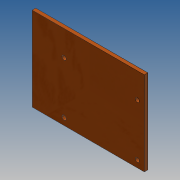
# Autodesk Inventor part: placa circuito
Saved by Autodesk Inventor 2017 (Build 210142000, 142)
## iProperties
Part Number: placa circuito
Material: Genérico
Document SubType Name: Modeling
Designer: Leo
Density: 1 g/cm^3
Appearance: Suave - Naranja claro
Author: Leo
Autodesk Inventor part; units mm, degrees
ref_plane "YZ Plane" through (0, 0, 0) normal (1, 0, 0) x (0, 1, 0)
ref_plane "XZ Plane" through (0, 0, 0) normal (0, 1, 0) x (-1, 0, 0)
ref_plane "XY Plane" through (0, 0, 0) normal (0, 0, 1) x (1, 0, 0)
sketch "Boceto1" plane through (0, 0, 0) normal (0, 1, 0) x (-1, 0, 0)
  line L0 (20, 30) -> (-76, 30)
  line L1 (-76, 30) -> (-76, -30)
  line L2 (-76, -30) -> (20, -30)
  line L3 (20, -30) -> (20, 30)
  line L4 (-3, -25) -> (-58, -25) construction
  line L5 (-58, -25) -> (-58, 15) construction
  line L6 (-58, 15) -> (-3, 15) construction
  line L7 (-3, 15) -> (-3, -25) construction
  circle A0 centre (-58, -25) radius 1.5
  circle A1 centre (-3, -25) radius 1.5
  circle A2 centre (-3, 15) radius 1.5
  circle A3 centre (-58, 15) radius 1.5
  point P0 (0, 0)
  point P1 (20, 0)
  dimension "d0" = 3
  dimension "d1" = 60
  dimension "d2" = 18
  dimension "d5" = 96
  dimension "d6" = 20
  dimension "d7" = 15
  dimension "d8" = 5
  dimension "d9" = 55
  constraints: 16 end point, 4 centre point, 4 coincident, 4 parallel, 3 equal radius, 2 perpendicular, 1 horizontal, 1 horizontal alignment, 1 midpoint
  measures "d0" diameter of A0
  measures "d1" distance of L2.end L0.start
  measures "d2" distance between parallel lines of L1 L5
  measures "d5" distance of L1.end L2.end
  measures "d6" distance from line of L3 point (0, 0)
  measures "d7" distance from line of point (0, 0) L6
  measures "d8" distance between parallel lines of L2 L4
  measures "d9" distance of L5.end L6.end
extrude "Extrusión1" add sketch "Boceto1" against normal blind 2.5
